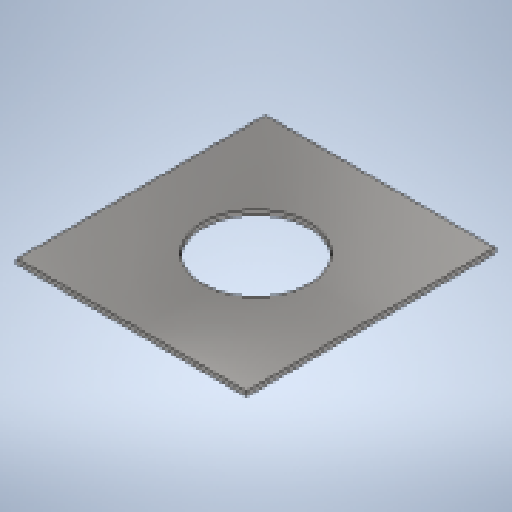
# Autodesk Inventor part: MSC 111 cone IN bottom
Saved by Autodesk Inventor 2025 (Build 290162010, 162A)
## iProperties
Created: 2024-05-19
Part Number: MSC 111 cone IN bottom
Material: Stainless Steel
Document SubType Name: Sheet Metal
Designer: admin
Density: 8 g/cm^3
Sheet Metal Rule: Default
Appearance: Semi-Polished
Stock Number: МОО 111 конус подача дно
Mass: 1076.42 g
Surface Area: 716.075 cm^2
Volume: 134.553 cm^3
Flat Pattern Width: 19.4 cm
Flat Pattern Length: 21.4 cm
Flat Pattern Area: 415.16 cm^2
Sheet Metal Width: 194,000 mm
Sheet Metal Length: 214,000 mm
Sheet Metal Area: 41516,000 mm^2
Конус_Угол_продольный: 52,40 deg
Конус_Угол_поперечный: 52,00 deg
Конус_Дно_сторона: 200,000 mm
Конус_ширина_по_оси: 1700,000 mm
Author: admin
Autodesk Inventor part; units mm, degrees
ref_plane "YZ Plane" through (0, 0, 0) normal (1, 0, 0) x (0, 1, 0)
ref_plane "XZ Plane" through (0, 0, 0) normal (0, 1, 0) x (-1, 0, 0)
ref_plane "XY Plane" through (0, 0, 0) normal (0, 0, 1) x (1, 0, 0)
sketch "Sketch1" plane through (0, 0, 0) normal (0, 0, 1) x (1, 0, 0)
  line L0 (-97, 107) -> (97, 107)
  line L1 (97, 107) -> (97, -107)
  line L2 (97, -107) -> (-97, -107)
  line L3 (-97, -107) -> (-97, 107)
  line L4 (-97, 107) -> (97, -107) construction
  line L5 (97, 107) -> (-97, -107) construction
  point P0 (0, 0)
  dimension "d0" = 194
  dimension "d1" = 214
  measures "d0" distance of L0.start L0.end
  measures "d1" distance of L0.end L1.end
extrude "Plate1" add sketch "Sketch1" along normal blind 4
sketch "Sketch2" plane through (0, 0, 0) normal (0, 0, 1) x (1, 0, 0)
  circle A0 centre (0, 0) radius 45
  dimension "d3" = 90
  constraints: 1 centre point, 1 coincident
  measures "d3" diameter of A0
extrude "Extrusion1" cut sketch "Sketch2" along normal blind 10
equation "\"d2\" = Thickness"
equation "\"BendRadius\" = Thickness"
equation "\"BendReliefWidth\" = Thickness"
equation "\"BendReliefDepth\" = 0.5 * Thickness"
equation "\"CornerReliefSize\" = 4 * Thickness"
equation "\"MinimumRemnant\" = 2 * Thickness"
equation "\"TransitionRadius\" = BendRadius"
equation "\"JacobiRadiusSize\" = BendRadius"
equation "\"GapSize\" = Thickness"
equation "\"Конус_Угол_продольный\" = 52.4deg"
equation "\"Конус_Угол_поперечный\" = 52deg"
equation "\"Thickness\" = 4"
body "Solid1"
